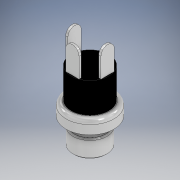
# Autodesk Inventor part: gniazdo_zasilania
Saved by Autodesk Inventor 2020 (Build 240168000, 168)
## iProperties
Created: 2020-11-28
Part Number: gniazdo_zasilania
Material: Generic
Document SubType Name: Modeling
Designer: Milosz
Density: 1 g/cm^3
Appearance: Default
Author: Milosz
Autodesk Inventor part; units mm, degrees
ref_plane "YZ Plane" through (0, 0, 0) normal (1, 0, 0) x (0, 1, 0)
ref_plane "XZ Plane" through (0, 0, 0) normal (0, 1, 0) x (-1, 0, 0)
ref_plane "XY Plane" through (0, 0, 0) normal (0, 0, 1) x (1, 0, 0)
sketch "Sketch1" plane through (0, 0, 0) normal (0, 1, 0) x (-1, 0, 0)
  circle A0 centre (0, 0) radius 5.4
  dimension "d0" = 10.8
  constraints: 1 centre point, 1 coincident
  measures "d0" diameter of A0
extrude "Extrusion1" add sketch "Sketch1" along normal blind 3
fillet "Fillet1" radius 1 1 edges at (5.4, 3, 0)
sketch "Sketch2" plane through (0, 3, 0) normal (0, 1, 0) x (1, 0, 0)
  circle A0 centre (0, 0) radius 4.25
  dimension "d4" = 8.5
  constraints: 1 centre point, 1 coincident
  measures "d4" diameter of A0
extrude "Extrusion2" add sketch "Sketch2" along normal blind 6.8
sketch "Sketch3" plane through (0, 0, 0) normal (0, -1, 0) x (1, 0, 0)
  circle A0 centre (0, 0) radius 3.5
  dimension "d7" = 7
  constraints: 1 centre point, 1 coincident
  measures "d7" diameter of A0
extrude "Extrusion3" add sketch "Sketch3" along normal blind 5.9
sketch "Sketch4" plane through (0, -5.9, 0) normal (0, -1, 0) x (1, 0, 0)
  circle A0 centre (0, 0) radius 4.25 projected
  circle A1 centre (0, 0) radius 3.83
  dimension "d10" = 7.66
  constraints: 1 centre point, 1 coincident
  measures "d10" diameter of A1
extrude "Extrusion4" add sketch "Sketch4" against normal blind 4 contours A1
sketch "Sketch5" plane through (0, 9.8, 0) normal (0, 1, 0) x (1, 0, 0)
  line L0 (-3.9765, 1.5) -> (-3.4765, 1.5)
  line L1 (-3.4765, 1.5) -> (-3.4765, -1.5)
  line L2 (-3.4765, -1.5) -> (-3.9765, -1.5)
  line L3 (-3.9765, -1.5) -> (-3.9765, 1.5)
  circle A0 centre (0, 0) radius 4.25 projected
  line L4 (-1.5, -3.9765) -> (-1.5, -3.4765)
  line L5 (-1.5, -3.4765) -> (1.5, -3.4765)
  line L6 (1.5, -3.4765) -> (1.5, -3.9765)
  line L7 (1.5, -3.9765) -> (-1.5, -3.9765)
  line L8 (3.9765, -1.5) -> (3.4765, -1.5)
  line L9 (3.4765, -1.5) -> (3.4765, 1.5)
  line L10 (3.4765, 1.5) -> (3.9765, 1.5)
  line L11 (3.9765, 1.5) -> (3.9765, -1.5)
  dimension "d13" = 0.5
  dimension "d14" = 3
  dimension "d17" = 180
  constraints: 24 end point, 2 parallel, 2 point on circle, 1 horizontal, 1 perpendicular, 17 other
  measures "d13" distance of L1.end L2.end
  measures "d14" distance of L0.end L1.end
extrude "Extrusion5" add sketch "Sketch5" along normal blind 6 contours L0 L1 L2 L3 | L11 L8 L9 L10 | L4 L5 L6 L7
fillet "Fillet2" radius 1.5 6 edges at (3.7265, 15.8, -1.5) (3.7265, 15.8, 1.5) (1.5, 15.8, 3.7265) (-1.5, 15.8, 3.7265) (-3.7265, 15.8, 1.5) (-3.7265, 15.8, -1.5)
chamfer "Chamfer1" distance 0.3 angle 45 1 edges at (-3.83, -1.9, 0)
chamfer "Chamfer2" distance 0.3 angle 45 1 edges at (-3.83, -5.9, 0)
sketch "Sketch6" plane through (0, -5.9, 0) normal (0, -1, 0) x (1, 0, 0)
  circle A0 centre (0, 0) radius 3.83 projected
  circle A1 centre (0, 0) radius 2.83
  dimension "d28" = 1
  constraints: 1 centre point
  measures "d28" radial gap between concentric circles of A0 A1
extrude "Extrusion6" cut sketch "Sketch6" against normal blind 8 contours A1
sketch "Sketch7" plane through (0, 2.1, 0) normal (0, -1, 0) x (1, 0, 0)
  circle A0 centre (0, 0) radius 1.1
  dimension "d31" = 2.2
  constraints: 1 centre point, 1 coincident
  measures "d31" diameter of A0
extrude "Extrusion7" add sketch "Sketch7" along normal blind 5.5
fillet "Fillet3" radius 1.1 1 edges at (-1.1, -3.4, 0)
equation "\"d34\" = 0.5 * d31"
body "Solid1"
